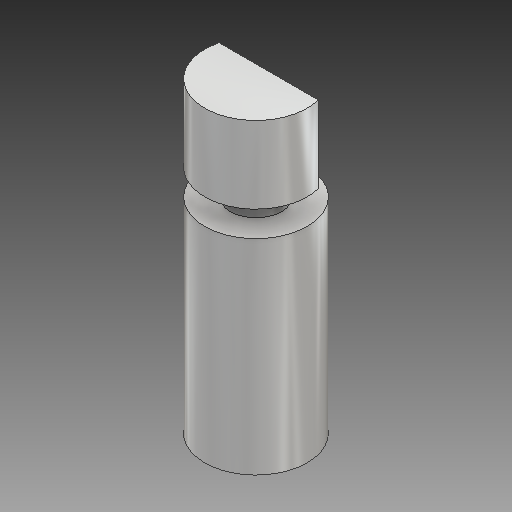
# Autodesk Inventor part: motor
Saved by Autodesk Inventor 2019 (Build 230136000, 136)
## iProperties
Created: 2016-09-25
Part Number: motor
Material: Aluminium 6061
Document SubType Name: Modeling
Designer: WhoTheHeck
Density: 2.7 g/cm^3
Appearance: Aluminium - poliert
Author: WhoTheHeck
Autodesk Inventor part; units mm, degrees
ref_plane "YZ Plane" through (0, 0, 0) normal (1, 0, 0) x (0, 1, 0)
ref_plane "XZ Plane" through (0, 0, 0) normal (0, 1, 0) x (-1, 0, 0)
sketch "Skizze1" plane through (0, 0, 0) normal (0, 0, 1) x (1, 0, 0)
  circle A0 centre (0, 0) radius 2
  dimension "d0" = 4
  constraints: 1 centre point, 1 coincident
  measures "d0" diameter of A0
extrude "Extrusion1" add sketch "Skizze1" along normal blind 12
sketch "Skizze2" plane through (0, 0, 12) normal (0, 0, 1) x (1, 0, 0)
  circle A0 centre (0, 0) radius 2 projected
  line L0 (-1.9372, 0.4972) -> (1.9372, 0.4972)
  constraints: 2 end point, 2 point on circle, 1 horizontal
extrude "Extrusion2" cut sketch "Skizze2" against normal blind 3 contours L0 A0 picked at (-0.0798, 0.9933)
ref_plane "Arbeitsebene1" through (0, 0, 9) normal (0, 0, 1) x (1, 0, 0)
sketch "Skizze3" plane through (0, 0, 9) normal (0, 0, 1) x (1, 0, 0)
  circle A0 centre (0, 0) radius 1
  arc A1 (1.9372, 0.4972) -> (-1.9372, 0.4972) centre (0, 0) ccw projected
  arc A2 (-1.9372, 0.4972) -> (1.9372, 0.4972) centre (0, 0) ccw projected
  dimension "d6" = 2
  constraints: 1 centre point, 1 coincident
  measures "d6" diameter of A0
extrude "Extrusion3" cut sketch "Skizze3" against normal blind 1
